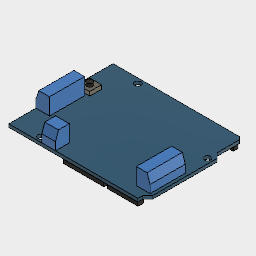
1438 Adafruit MotorShield V2 (Autodesk Fusion 360 design; units mm, degrees)
Autodesk Fusion 360 part; units mm, degrees
sketch "Adafruit Motor Shield v2.3" plane through (0, 0, 0) normal (0, 0, 1) x (1, 0, 0)
  line L0 (0, 53.34) -> (64.516, 53.34)
  line L1 (0, 0) -> (66.04, 0)
  line L2 (64.516, 53.34) -> (66.04, 51.816)
  circle A0 centre (15.24, 50.8) radius 1.6
  line L3 (66.04, 2.54) -> (66.04, 0)
  line L4 (66.04, 51.816) -> (64.516, 53.34)
  line L5 (66.04, 2.54) -> (68.58, 5.08)
  circle A1 centre (13.97, 2.54) radius 1.6
  line L6 (64.516, 53.34) -> (0, 53.34)
  line L7 (68.58, 5.08) -> (68.58, 37.846)
  line L8 (66.04, 51.816) -> (66.04, 40.386)
  line L9 (66.04, 40.386) -> (68.58, 37.846)
  circle A2 centre (66.04, 35.56) radius 1.6
  line L10 (0, 53.34) -> (0, 0)
  line L11 (68.58, 37.846) -> (66.04, 40.386)
  line L12 (68.58, 5.08) -> (66.04, 2.54)
  line L13 (68.58, 37.846) -> (68.58, 5.08)
  line L14 (66.04, 0) -> (0, 0)
  line L15 (0, 0) -> (0, 53.34)
  line L16 (66.04, 0) -> (66.04, 2.54)
  line L17 (66.04, 40.386) -> (66.04, 51.816)
extrude "Extrude1" add sketch "Adafruit Motor Shield v2.3" along normal blind 1.64 makes body 1
sketch "Sketch2" plane through (0, 0, 1.64) normal (0, 0, 1) x (-1, 0, 0)
  circle A0 centre (-13.97, -2.54) radius 1.6
  circle A1 centre (-15.24, -50.8) radius 1.6
  circle A2 centre (-66.04, -35.56) radius 1.6
  line L0 (-68.58, -37.846) -> (-66.04, -40.386)
  line L1 (-66.04, -40.386) -> (-66.04, -51.816)
  line L2 (-66.04, -51.816) -> (-64.516, -53.34)
  line L3 (-64.516, -53.34) -> (0, -53.34)
  line L4 (0, -53.34) -> (0, 0)
  line L5 (0, 0) -> (-66.04, 0)
  line L6 (-66.04, 0) -> (-66.04, -2.54)
  line L7 (-66.04, -2.54) -> (-68.58, -5.08)
  line L8 (-68.58, -5.08) -> (-68.58, -37.846)
  line L9 (0, -31.86) -> (-7, -31.86)
  line L10 (-7, -31.86) -> (-7, -13.86)
  line L11 (-7, -13.86) -> (0, -13.86)
  line L12 (0, -13.86) -> (0, -31.86)
  line L13 (-23.947, 0) -> (-16.947, 0)
  line L14 (-16.947, 0) -> (-16.947, -7)
  line L15 (-16.947, -7) -> (-23.947, -7)
  line L16 (-23.947, -7) -> (-23.947, 0)
  line L17 (-23.947, 0) -> (-16.947, -7) construction
  line L18 (-16.947, 0) -> (-23.947, -7) construction
  line L19 (-7, -22.86) -> (0, -22.86) construction
  line L20 (-60, -23.224) -> (-67, -23.224)
  line L21 (-67, -23.224) -> (-67, -5.224)
  line L22 (-67, -5.224) -> (-60, -5.224)
  line L23 (-60, -5.224) -> (-60, -23.224)
  line L24 (-67, -14.224) -> (-60, -14.224) construction
  point P0 (-20.447, -3.5)
  dimension "d3" = 18
  dimension "d4" = 7
  dimension "d7" = 7
  dimension "d8" = 7
  dimension "d9" = 20.447
  dimension "d10" = 22.86
  dimension "d11" = 7
  dimension "d12" = 18
  dimension "d13" = 14.224
  measures "d3" distance of L9.start L11.end
  measures "d4" distance of L9.start L9.end
  measures "d7" distance of L13.end L14.end
  measures "d8" distance of L14.end L15.end
  measures "d9" distance of L4 P0
  measures "d10" distance of L5 L19
  measures "d11" distance of L20.start L20.end
  measures "d12" distance of L20.start L22.end
  measures "d13" distance of L5 L24
extrude "Extrude2" add sketch "Sketch2" along normal blind 4 separate body contours L5 L13 L14 L15 L16 | L4 L9 L10 L11 L12 | L20 L21 L22 L23 makes body 2 at (4.6667, 25.86, 1.64) makes body 3 at (21.6137, 2.3333, 1.64) makes body 4 at (62.3333, 17.224, 1.64)
sketch "Sketch3" plane through (0, 0, 5.64) normal (0, 0, 1) x (-1, 0, 0)
  line L0 (0, -13.86) -> (-7, -13.86)
  line L1 (-7, -13.86) -> (-7, -31.86)
  line L2 (-7, -31.86) -> (0, -31.86)
  line L3 (0, -31.86) -> (0, -13.86)
  line L4 (-60, -5.224) -> (-67, -5.224)
  line L5 (-67, -5.224) -> (-67, -23.224)
  line L6 (-67, -23.224) -> (-60, -23.224)
  line L7 (-60, -23.224) -> (-60, -5.224)
  line L8 (-23.947, -7) -> (-16.947, -7)
  line L9 (-16.947, -7) -> (-16.947, 0)
  line L10 (-16.947, 0) -> (-23.947, 0)
  line L11 (-23.947, 0) -> (-23.947, -7)
  line L12 (-7, -31.86) -> (-1.5, -31.86)
  line L13 (-1.5, -31.86) -> (-1.5, -13.86)
  line L14 (-1.5, -13.86) -> (-7, -13.86)
  line L15 (-7, -13.86) -> (-7, -31.86)
  line L16 (-23.947, -7) -> (-16.947, -7)
  line L17 (-16.947, -7) -> (-16.947, -1.5)
  line L18 (-16.947, -1.5) -> (-23.947, -1.5)
  line L19 (-23.947, -1.5) -> (-23.947, -7)
  line L20 (-60, -5.224) -> (-65.5, -5.224)
  line L21 (-65.5, -5.224) -> (-65.5, -23.224)
  line L22 (-65.5, -23.224) -> (-60, -23.224)
  line L23 (-60, -23.224) -> (-60, -5.224)
  dimension "d16" = 5.5
  dimension "d17" = 18
  dimension "d18" = 5.5
  dimension "d19" = 7
  dimension "d20" = 5.5
  dimension "d21" = 18
  measures "d16" distance of L1.end L12.end
  measures "d17" distance of L1.end L0.end
  measures "d18" distance of L8.start L18.end
  measures "d19" distance of L8.start L8.end
  measures "d20" distance of L4.start L20.end
  measures "d21" distance of L4.start L6.end
extrude "Extrude3" add sketch "Sketch3" along normal blind 4.5 contours L0 L1 L2 L12 L13 L14 L15 | L4 L6 L7 L20 L21 L22 L23 | L8 L9 L11 L16 L17 L18 L19 bodies 2 3 4
draft "Draft1" angle 18.5 neutral plane through (0, 0, 10.14) pull (0, 0, 1) 1 faces at (1.5, 25.86, 7.14) on bodies 2
draft "Draft2" angle 18.5 neutral plane through (0, 0, 10.14) pull (0, 0, 1) 1 faces at (19.2803, 1.5, 7.14) on bodies 3
draft "Draft3" angle 18.5 neutral plane through (0, 0, 10.14) pull (0, 0, 1) 1 faces at (65.5, 11.224, 7.14) on bodies 4
sketch "Sketch4" plane through (0, 0, 1.64) normal (0, 0, 1) x (-1, 0, 0)
  circle A0 centre (-13.97, -2.54) radius 1.6
  circle A1 centre (-15.24, -50.8) radius 1.6
  circle A2 centre (-66.04, -35.56) radius 1.6
  line L0 (-68.58, -37.846) -> (-66.04, -40.386)
  line L1 (-66.04, -40.386) -> (-66.04, -51.816)
  line L2 (-66.04, -51.816) -> (-64.516, -53.34)
  line L3 (-64.516, -53.34) -> (0, -53.34)
  line L4 (0, -53.34) -> (0, 0)
  line L5 (0, 0) -> (-66.04, 0)
  line L6 (-66.04, 0) -> (-66.04, -2.54)
  line L7 (-66.04, -2.54) -> (-68.58, -5.08)
  line L8 (-68.58, -5.08) -> (-68.58, -37.846)
  line L9 (-49.24, -4.1) -> (-64.94, -4.1)
  line L10 (-64.94, -4.1) -> (-64.94, -1.1)
  line L11 (-64.94, -1.1) -> (-49.24, -1.1)
  line L12 (-49.24, -1.1) -> (-49.24, -4.1)
  line L13 (-47.6657, -4) -> (-26.8657, -4)
  line L14 (-26.8657, -4) -> (-26.8657, -1)
  line L15 (-26.8657, -1) -> (-47.6657, -1)
  line L16 (-47.6657, -1) -> (-47.6657, -4)
  line L17 (-64.94, -52.24) -> (-44.14, -52.24)
  line L18 (-44.14, -52.24) -> (-44.14, -49.74)
  line L19 (-44.14, -49.74) -> (-64.94, -49.74)
  line L20 (-64.94, -49.74) -> (-64.94, -52.24)
  line L21 (-43.14, -52.24) -> (-17.29, -52.24)
  line L22 (-17.29, -52.24) -> (-17.29, -49.74)
  line L23 (-17.29, -49.74) -> (-43.14, -49.74)
  line L24 (-43.14, -49.74) -> (-43.14, -52.24)
  dimension "d30" = 3
  dimension "d31" = 15.7
  dimension "d32" = 1.1
  dimension "d33" = 1.1
  dimension "d34" = 20.8
  dimension "d35" = 20.8
  dimension "d36" = 2.5
  dimension "d37" = 25.85
  dimension "d38" = 1
  dimension "d39" = 1.1
  dimension "d40" = 1.1
  measures "d30" distance of L9.end L10.end
  measures "d31" distance of L9.start L9.end
  measures "d32" distance of L6 L10
  measures "d33" distance of L5 L11
  measures "d34" distance of L13.start L13.end
  measures "d35" distance of L17.start L17.end
  measures "d36" distance of L17.start L19.end
  measures "d37" distance of L21.start L21.end
  measures "d38" distance of L18 L24
  measures "d39" distance of L1 L20
  measures "d40" distance of L3 L17
extrude "Extrude4" add sketch "Sketch4" against normal blind 3 from surface at -1.64 separate body contours L9 L10 L11 L12 | L13 L14 L15 L16 | L17 L18 L19 L20 | L21 L22 L23 L24 makes body 5 at (51.0733, 49.74, -1) makes body 6 at (59.7067, 2.1, 0) makes body 7 at (25.9067, 49.74, -1) makes body 8 at (40.7324, 3, 0)
sketch "Sketch5" plane through (0, 0, 1.64) normal (0, 0, 1) x (-1, 0, 0)
  circle A0 centre (-13.97, -2.54) radius 1.6
  circle A1 centre (-15.24, -50.8) radius 1.6
  circle A2 centre (-66.04, -35.56) radius 1.6
  line L0 (-68.58, -37.846) -> (-66.04, -40.386)
  line L1 (-66.04, -40.386) -> (-66.04, -51.816)
  line L2 (-66.04, -51.816) -> (-64.516, -53.34)
  line L3 (-64.516, -53.34) -> (0, -53.34)
  line L4 (0, -53.34) -> (0, 0)
  line L5 (0, 0) -> (-66.04, 0)
  line L6 (-66.04, 0) -> (-66.04, -2.54)
  line L7 (-66.04, -2.54) -> (-68.58, -5.08)
  line L8 (-68.58, -5.08) -> (-68.58, -37.846)
  line L9 (-8.461, -32.941) -> (-2.461, -32.941)
  line L10 (-2.461, -32.941) -> (-2.461, -38.941)
  line L11 (-2.461, -38.941) -> (-8.461, -38.941)
  line L12 (-8.461, -38.941) -> (-8.461, -32.941)
  line L13 (-8.461, -32.941) -> (-2.461, -38.941) construction
  line L14 (-2.461, -32.941) -> (-8.461, -38.941) construction
  circle A3 centre (-5.461, -35.941) radius 1.5
  point P0 (-5.461, -35.941)
  dimension "d44" = 6
  dimension "d45" = 6
  dimension "d46" = 3
  dimension "d47" = 5.461
  dimension "d48" = 35.941
  measures "d44" distance of L10.end L11.end
  measures "d45" distance of L9.end L10.end
  measures "d46" diameter of A3
  measures "d47" distance of L4 P0
  measures "d48" distance of L5 P0
extrude "Extrude5" add sketch "Sketch5" along normal blind 2 separate body contours L9 L10 L11 L12 | A3 makes body 9
extrude "Extrude6" add sketch "Sketch5" along normal blind 1.5 from surface at 2 contours A3 bodies 9
named bodies: "PCB", "button"
